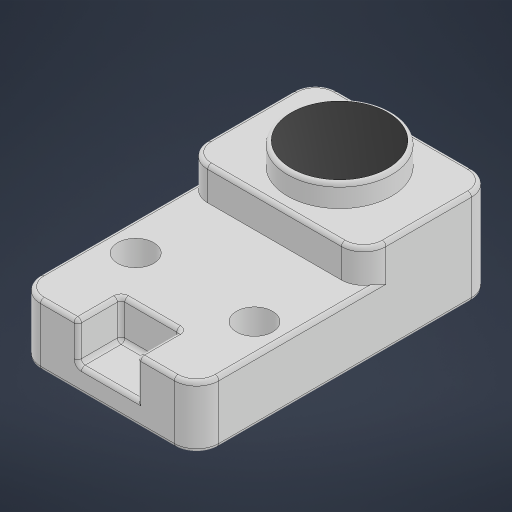
# Autodesk Inventor part: UnitV_OV7740_M12
Saved by Autodesk Inventor 2024.2 (Build 282272000, 272)
## iProperties
Created: 2023-12-21
Part Number: UnitV_OV7740_M12
Material: 一般
Document SubType Name: Modeling
Designer: Hanaoka
Density: 1 g/cm^3
Appearance: 既定
Author: Hanaoka
Autodesk Inventor part; units mm, degrees
ref_plane "YZ Plane" through (0, 0, 0) normal (1, 0, 0) x (0, 1, 0)
ref_plane "XZ Plane" through (0, 0, 0) normal (0, 1, 0) x (-1, 0, 0)
ref_plane "XY Plane" through (0, 0, 0) normal (0, 0, 1) x (1, 0, 0)
sketch "スケッチ1" plane through (0, 0, 0) normal (0, 1, 0) x (-1, 0, 0)
  line L0 (-9, 20) -> (9, 20)
  line L1 (12, 17) -> (12, -17)
  line L2 (9, -20) -> (-9, -20)
  line L3 (-12, -17) -> (-12, 17)
  line L4 (-12, 20) -> (12, -20) construction
  line L5 (12, 20) -> (-12, -20) construction
  line L6 (0, -28.8698) -> (0, 28.8698) projected
  circle A0 centre (8, 8.2) radius 2.425
  circle A1 centre (-8, 8.2) radius 2.425
  arc A2 (12, 17) -> (9, 20) centre (9, 17) ccw
  arc A3 (-9, 20) -> (-12, 17) centre (-9, 17) ccw
  arc A4 (-12, -17) -> (-9, -20) centre (-9, -17) ccw
  arc A5 (9, -20) -> (12, -17) centre (9, -17) ccw
  point P0 (0, 0)
  dimension "d0" = 24
  dimension "d1" = 40
  dimension "d4" = 4.85
  dimension "d5" = 16
  dimension "d6" = 11.8
  dimension "d7" = 3
  constraints: 12 end point, 8 point on circle, 8 point on line, 8 tangent, 6 centre point, 4 equal radius, 2 midpoint, 2 parallel, 1 horizontal, 1 horizontal alignment, 1 perpendicular, 1 other
  measures "d0" distance of L4.end L5.end
  measures "d1" distance of L5.start L4.end
  measures "d4" diameter of A0
  measures "d5" distance of A1.centre A0.centre
  measures "d6" distance from line of L0 A0.centre
  measures "d7" radius of A2
extrude "押し出し1" add sketch "スケッチ1" along normal blind 8.3
sketch "スケッチ2" plane through (0, 8.3, 0) normal (0, 1, 0) x (1, 0, 0)
  line L0 (-12, 17) -> (-12, -17) projected
  line L1 (-9, 2.5) -> (9, 2.5)
  line L2 (12, -17) -> (12, 17) projected
  line L3 (-12, 17) -> (-12, 5.5)
  line L4 (12, 17) -> (12, 5.5)
  arc A0 (-12, 5.5) -> (-9, 2.5) centre (-9, 5.5) ccw
  arc A1 (9, 2.5) -> (12, 5.5) centre (9, 5.5) ccw
  line L5 (9, 20) -> (-9, 20) projected
  arc A2 (-9, 20) -> (-12, 17) centre (-9, 17) ccw projected
  arc A3 (12, 17) -> (9, 20) centre (9, 17) ccw projected
  point P0 (0, 0)
  point P1 (-12, 2.5)
  point P2 (12, 2.5)
  dimension "d10" = 3
  dimension "d11" = 17.5
  constraints: 6 end point, 6 point on line, 4 point on circle, 4 tangent, 2 centre point, 1 equal radius, 1 horizontal, 1 parallel, 1 perpendicular
  measures "d10" radius of A0
  measures "d11" distance between parallel lines of L5 L1
extrude "押し出し2" add sketch "スケッチ2" along normal blind 4.4
sketch "スケッチ3" plane through (0, 12.7, 0) normal (0, 1, 0) x (1, 0, 0)
  circle A0 centre (0, 11.25) radius 7
  line L0 (-12, 17) -> (-12, 5.5) projected
  line L1 (-12, 11.25) -> (12, 11.25) construction
  line L2 (12, 5.5) -> (12, 17) projected
  line L3 (9, 20) -> (-9, 20) projected
  line L4 (0, 20) -> (0, 2.5) construction
  line L5 (-9, 2.5) -> (9, 2.5) projected
  point P0 (0, 0)
  dimension "d14" = 14
  constraints: 5 midpoint, 4 end point, 1 centre point, 1 coincident, 1 vertical
  measures "d14" diameter of A0
extrude "押し出し3" add sketch "スケッチ3" along normal blind 3
fillet "フィレット1" radius 0.5 1 edges at (-7, 15.7, -11.25)
fillet "フィレット2" radius 0.5 21 edges at (11.1213, 8.3, 19.1213) (0, 8.3, 20) (-11.1213, 8.3, 19.1213) (-12, 8.3, 5.75) (12, 8.3, 5.75) (11.1213, 12.7, -3.3787) (12, 12.7, -11.25) (11.1213, 12.7, -19.1213) (0, 12.7, -20) (-11.1213, 12.7, -19.1213) (-12, 12.7, -11.25) (-11.1213, 12.7, -3.3787) (0, 12.7, -2.5) (11.1213, 0, 19.1213) (12, 0, 0) (11.1213, 0, -19.1213) (0, 0, -20) (-11.1213, 0, -19.1213) (-12, 0, 0) (-11.1213, 0, 19.1213) (0, 0, 20)
sketch "スケッチ4" plane through (0, 0, 0) normal (1, 0, 0) x (0, 1, 0)
  line L0 (10.3657, 22.992) -> (3.1274, 22.992)
  line L1 (3.1274, 22.992) -> (3.1274, 14.1637)
  line L2 (3.1274, 14.1637) -> (10.3657, 14.1637)
  line L3 (10.3657, 14.1637) -> (10.3657, 22.992)
  point P0 (0, 0)
  constraints: 8 end point, 2 parallel, 1 horizontal, 1 perpendicular
extrude "押し出し4" cut sketch "スケッチ4" along normal mid plane 8
fillet "フィレット3" radius 0.5 12 edges at (0, 8.3, 14.1637) (-4, 8.1536, 19.8536) (-4, 5.4637, 20) (-4, 8.3, 16.8319) (-4, 5.7137, 14.1637) (-4, 3.1274, 17.0819) (0, 3.1274, 14.1637) (4, 8.1536, 19.8536) (4, 8.3, 16.8319) (4, 5.4637, 20) (0, 3.1274, 20) (4, 5.7137, 14.1637)
